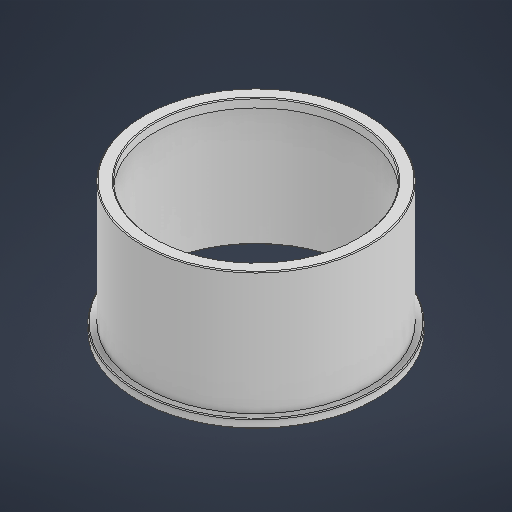
# Autodesk Inventor part: Cylinder  Segment - 08
Saved by Autodesk Inventor 2025 (Build 290162000, 162)
## iProperties
Created: 2024-04-11
Part Number: Cylinder  Segment - 08
Material: Generic
Document SubType Name: Modeling
Designer: Thienan Hoang
Density: 1 g/cm^3
Appearance: Default
Author: Thienan Hoang
Autodesk Inventor part; units mm, degrees
ref_plane "YZ Plane" through (0, 0, 0) normal (1, 0, 0) x (0, 1, 0)
ref_plane "XZ Plane" through (0, 0, 0) normal (0, 1, 0) x (-1, 0, 0)
ref_plane "XY Plane" through (0, 0, 0) normal (0, 0, 1) x (1, 0, 0)
sketch "Sketch1" plane through (0, 0, 0) normal (0, 1, 0) x (-1, 0, 0)
  circle A0 centre (0, 0) radius 67.875
  circle A1 centre (0, 0) radius 64.25
  circle A2 centre (0, 0) radius 61.125
  circle A3 centre (0, 0) radius 9.5
  dimension "Absolute_Diameter" = 135.75
  dimension "Diameter_No_Outer_Lip" = 128.5
  dimension "Inner_Cylinder_Diameter" = 122.25
  dimension "Lip_Diameter" = 19
  constraints: 4 centre point, 4 coincident
  measures "Absolute_Diameter" diameter of A0
  measures "Diameter_No_Outer_Lip" diameter of A1
  measures "Inner_Cylinder_Diameter" diameter of A2
  measures "Lip_Diameter" diameter of A3
extrude "Extrusion1" add sketch "Sketch1" along normal blind 5 contours A0
extrude "Extrusion2" add sketch "Sketch1" along normal blind 75 contours A1
sketch "Sketch2" plane through (0, 75, 0) normal (0, 1, 0) x (1, 0, 0)
  circle A0 centre (0, 0) radius 64.25
  circle A1 centre (0, 0) radius 57.5
  dimension "Lip_Diameter_Out" = 128.5
  dimension "Inner_Lip_Diameter" = 115
  constraints: 2 centre point, 1 coincident
  measures "Lip_Diameter_Out" diameter of A0
  measures "Inner_Lip_Diameter" diameter of A1
extrude "Extrusion7" add sketch "Sketch2" against normal blind 5
chamfer "Chamfer1" distance 0.5 angle 45 2 edges at (64.25, 75, 0) (-57.5, 75, 0)
chamfer "Chamfer2" distance 0.5 angle 45 3 edges at (67.875, 5, 0) (67.875, 0, 0) (61.125, 0, 0)
sketch "Sketch3" plane through (0, 5, 0) normal (0, 1, 0) x (1, 0, 0)
  circle A0 centre (0, 0) radius 127.5
  circle A1 centre (-127.5, 0) radius 2
  circle A2 centre (-103.1497, -74.9426) radius 2
  circle A3 centre (-39.3997, -121.2597) radius 2
  circle A4 centre (39.3997, -121.2597) radius 2
  circle A5 centre (103.1497, -74.9426) radius 2
  circle A6 centre (127.5, 0) radius 2
  circle A7 centre (103.1497, 74.9426) radius 2
  circle A8 centre (39.3997, 121.2597) radius 2
  circle A9 centre (-39.3997, 121.2597) radius 2
  circle A10 centre (-103.1497, 74.9426) radius 2
  dimension "d27" = 255
  dimension "d28" = 4
  dimension "d31" = 360
  constraints: 10 centre point, 1 coincident, 1 horizontal alignment, 23 other
  measures "d28" diameter of A1
extrude "Extrusion8" [suppressed]
sketch "Sketch4" plane through (0, 75, 0) normal (0, 1, 0) x (1, 0, 0)
  circle A0 centre (0, 0) radius 42.5
  circle A1 centre (0, 0) radius 37.5
  circle A2 centre (0, 0) radius 40
  circle A3 centre (-40, 0) radius 1
  circle A4 centre (-24.9396, -31.2733) radius 1
  circle A5 centre (8.9008, -38.9971) radius 1
  circle A6 centre (36.0388, -17.3553) radius 1
  circle A7 centre (36.0388, 17.3553) radius 1
  circle A8 centre (8.9008, 38.9971) radius 1
  circle A9 centre (-24.9396, 31.2733) radius 1
  dimension "d35" = 80
  dimension "d36" = 2
  dimension "d39" = 360
  constraints: 9 centre point, 3 coincident, 1 horizontal alignment, 17 other
  measures "d36" diameter of A3
hole "Hole1" [suppressed]
body "Solid1"
